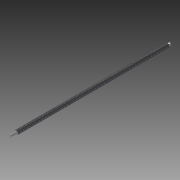
# Autodesk Inventor part: Z Axis Lead Screw
Saved by Autodesk Inventor 2015 SP1 (Build 190203100, 203)
## iProperties
Category: Hardware
Material: Steel
Document SubType Name: Modeling
Designer: Jack
Density: 7.85 g/cm^3
Appearance: Steel
Mass: 120.995 g
Surface Area: 79.0739 cm^2
Volume: 15.4134 cm^3
Vendor: MakersToolWorks
Author: Jack
Title: Z Axis Lead Screw
Autodesk Inventor part; units mm, degrees
ref_plane "YZ Plane" through (0, 0, 0) normal (1, 0, 0) x (0, 1, 0)
ref_plane "XZ Plane" through (0, 0, 0) normal (0, 1, 0) x (-1, 0, 0)
ref_plane "XY Plane" through (0, 0, 0) normal (0, 0, 1) x (1, 0, 0)
sketch "Sketch1" plane through (0, 0, 0) normal (0, 1, 0) x (-1, 0, 0)
  circle A0 centre (0, 0) radius 2.5
  dimension "d0" = 5
  constraints: 1 centre point, 1 coincident
  measures "d0" diameter of A0
extrude "Extrusion1" add sketch "Sketch1" along normal blind 12
sketch "Sketch5" plane through (0, 12, 0) normal (0, 1, 0) x (1, 0, 0)
  circle A0 centre (0, 0) radius 2.5 projected
  circle A1 centre (0, 0) radius 4
  dimension "d20" = 8
  constraints: 1 centre point, 1 coincident
  measures "d20" diameter of A1
extrude "Extrusion5" add sketch "Sketch5" along normal blind 300 contours A0 | A1
sketch "Sketch6" plane through (0, 312, 0) normal (0, 1, 0) x (1, 0, 0)
  circle A0 centre (0, 0) radius 4 projected
  circle A1 centre (0, 0) radius 2.5
  dimension "d23" = 5
  constraints: 1 centre point, 1 coincident
  measures "d23" diameter of A1
extrude "Extrusion6" add sketch "Sketch6" along normal blind 5 contours A1
thread "Thread2" size "M10x1.5" class "6g" standard "ANSI Metric M Profile" full length
thread "Thread3" size "TR10x1.5" class "7e" standard "ISO Metric Trapezoidal Threads" full length
body "Solid1"
